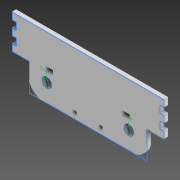
# Autodesk Inventor part: Zijkant
Saved by Autodesk Inventor 2020.2 (Build 242310000, 310)
## iProperties
Created: 2020-05-21
Part Number: Zijkant
Material: Generic
Document SubType Name: Modeling
Designer: Berkant
Density: 1 g/cm^3
Appearance: Default
Author: Berkant
Autodesk Inventor part; units mm, degrees
ref_plane "YZ Plane" through (0, 0, 0) normal (1, 0, 0) x (0, 1, 0)
ref_plane "XZ Plane" through (0, 0, 0) normal (0, 1, 0) x (-1, 0, 0)
ref_plane "XY Plane" through (0, 0, 0) normal (0, 0, 1) x (1, 0, 0)
sketch "Sketch1" plane through (0, 0, 0) normal (0, 0, 1) x (1, 0, 0)
  line L0 (12.5, 0) -> (98.5, 0)
  line L1 (111, 45) -> (0, 45)
  line L2 (12.5, 20) -> (12.5, 0)
  line L3 (111, 20) -> (98.5, 20) construction
  line L4 (111, 20) -> (98.5, 20)
  line L5 (98.5, 20) -> (98.5, 0)
  line L6 (12.5, 20) -> (0, 20)
  line L7 (12.5, 0) -> (25.5, 0) construction
  line L8 (12.5, 13) -> (12.5, 0) construction
  line L9 (98.5, 0) -> (85.5, 0) construction
  line L10 (98.5, 13) -> (98.5, 0) construction
  line L11 (0, 45) -> (0, 40)
  line L12 (0, 40) -> (3, 40)
  line L13 (3, 40) -> (3, 35)
  line L14 (3, 35) -> (0, 35)
  line L15 (0, 35) -> (0, 30)
  line L16 (0, 30) -> (3, 30)
  line L17 (3, 30) -> (3, 25)
  line L18 (3, 25) -> (0, 25)
  line L19 (0, 25) -> (0, 20)
  line L20 (0, 45) -> (0, 40)
  line L21 (0, 35) -> (0, 30)
  line L22 (0, 25) -> (0, 20)
  line L23 (111, 45) -> (111, 40)
  line L24 (111, 40) -> (108, 40)
  line L25 (108, 40) -> (108, 35)
  line L26 (108, 35) -> (111, 35)
  line L27 (111, 35) -> (111, 30)
  line L28 (111, 30) -> (108, 30)
  line L29 (108, 30) -> (108, 25)
  line L30 (108, 25) -> (111, 25)
  line L31 (111, 25) -> (111, 20)
  line L32 (111, 40) -> (111, 45)
  line L33 (111, 20) -> (111, 25)
  line L34 (111, 30) -> (111, 35)
  circle A0 centre (25.5, 13) radius 3.5
  circle A1 centre (85.5, 13) radius 3.5
  dimension "d52" = 7
  dimension "d53" = 7
  constraints: 70 end point, 7 perpendicular, 4 horizontal, 4 point on line, 3 vertical, 2 centre point, 1 parallel
  measures "d52" diameter of A0
  measures "d53" diameter of A1
extrude "Extrusion1" add sketch "Sketch1" against normal blind 3 contours L2 L6 L19 L18 L17 L16 L15 L14 L13 L12 L11 L1 L23 L24 L25 L26 L27 L28 L29 L30 L31 L4 L5 L0 | A0 | A1
fillet "Fillet1" radius 10 2 edges at (12.5, 0, -1.5) (98.5, 0, -1.5)
sketch "Sketch2" plane through (0, 0, 0) normal (0, 0, 1) x (1, 0, 0)
  line L0 (25, 20) -> (30, 20)
  line L1 (30, 20) -> (30, 23)
  line L2 (30, 23) -> (25, 23)
  line L3 (25, 23) -> (25, 20)
  line L4 (86, 20) -> (81, 20)
  line L5 (81, 20) -> (81, 23)
  line L6 (81, 23) -> (86, 23)
  line L7 (86, 23) -> (86, 20)
  point P0 (0, 0)
  point P1 (0, 20)
  point P2 (111, 20)
  dimension "d32" = 5
  dimension "d33" = 3
  dimension "d34" = 5
  dimension "d35" = 25
  dimension "d36" = 5
  dimension "d37" = 3
  dimension "d38" = 5
  constraints: 16 end point, 4 perpendicular
  measures "d32" distance of L0.start L0.end
  measures "d33" distance of L0.end L1.end
  measures "d34" distance of L1.end L2.end
  measures "d35" distance of point (111, 20) L4.start
  measures "d36" distance of L4.start L4.end
  measures "d37" distance of L4.end L5.end
  measures "d38" distance of L5.end L6.end
extrude "Extrusion3" cut sketch "Sketch2" against normal blind 10
sketch "Sketch3" plane through (0, 0, 0) normal (0, 0, 1) x (1, 0, 0)
  circle A0 centre (64.9, 4.25) radius 1.5
  line L0 (0, 45) -> (111, 45) projected
  circle A1 centre (46.1, 4.25) radius 1.5
  point P0 (0, 0)
  point P1 (85.5, 13)
  dimension "d49" = 3
  dimension "d50" = 3
  constraints: 2 centre point
  measures "d49" diameter of A1
  measures "d50" diameter of A0
extrude "Extrusion4" cut sketch "Sketch3" against normal blind 10
extrude "Extrusion5" cut sketch "Sketch1" against normal blind 10 contours A0 | A1
body "Solid1"
